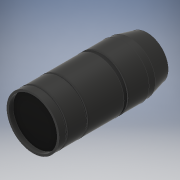
# Autodesk Inventor part: MLM3X-MP
Saved by Autodesk Inventor 2019 (Build 230136000, 136)
## iProperties
Created: 2019-03-17
Part Number: MLM3X-MP
Material: Acetal Resin, Black
Document SubType Name: Modeling
Designer: Wilson Lab
Density: 1.425 g/cm^3
Appearance: Smooth - Black
Author: Wilson Lab
Autodesk Inventor part; units mm, degrees
ref_plane "YZ Plane" through (0, 0, 0) normal (1, 0, 0) x (0, 1, 0)
ref_plane "XZ Plane" through (0, 0, 0) normal (0, 1, 0) x (-1, 0, 0)
ref_plane "XY Plane" through (0, 0, 0) normal (0, 0, 1) x (1, 0, 0)
sketch "Sketch1" plane through (0, 0, 0) normal (0, 0, 1) x (1, 0, 0)
  circle A0 centre (0, 0) radius 17.75
  dimension "d0" = 35.5
  constraints: 1 centre point, 1 coincident
  measures "d0" diameter of A0
extrude "Extrusion1" add sketch "Sketch1" along normal blind 16.8
sketch "Sketch2" plane through (0, 0, 16.8) normal (0, 0, 1) x (1, 0, 0)
  circle A0 centre (0, 0) radius 17.75 projected
  circle A1 centre (0, 0) radius 18.25
  dimension "d3" = 36.5
  constraints: 1 centre point, 1 coincident
  measures "d3" diameter of A1
extrude "Extrusion2" add sketch "Sketch2" along normal blind 14.7 contours A0 | A1
chamfer "Chamfer1" distance 3 distance2 12 1 edges at (-17.75, 0, 0) measured on face at (-0.7132, -5.1908, 0)
sketch "Sketch3" plane through (0, 0, 31.5) normal (0, 0, 1) x (1, 0, 0)
  circle A0 centre (0, 0) radius 18.25 projected
  circle A1 centre (0, 0) radius 17.75
  dimension "d9" = 35.5
  constraints: 1 centre point, 1 coincident
  measures "d9" diameter of A1
extrude "Extrusion3" add sketch "Sketch3" along normal blind 2.8 contours A1
sketch "Sketch4" plane through (0, 0, 34.3) normal (0, 0, 1) x (1, 0, 0)
  circle A0 centre (0, 0) radius 17.75 projected
  circle A1 centre (0, 0) radius 18.25
  dimension "d12" = 36.5
  constraints: 1 centre point, 1 coincident
  measures "d12" diameter of A1
extrude "Extrusion4" add sketch "Sketch4" along normal blind 25.25 contours A0 | A1
sketch "Sketch5" plane through (0, 0, 59.55) normal (0, 0, 1) x (1, 0, 0)
  circle A0 centre (0, 0) radius 18.25 projected
  circle A1 centre (0, 0) radius 17.75
  dimension "d15" = 35.5
  constraints: 1 centre point, 1 coincident
  measures "d15" diameter of A1
extrude "Extrusion5" add sketch "Sketch5" along normal blind 1 contours A1
sketch "Sketch6" plane through (0, 0, 60.55) normal (0, 0, 1) x (1, 0, 0)
  circle A0 centre (0, 0) radius 17.75 projected
  circle A1 centre (0, 0) radius 18.25
  dimension "d18" = 36.5
  constraints: 1 centre point, 1 coincident
  measures "d18" diameter of A1
extrude "Extrusion6" add sketch "Sketch6" along normal blind 13.2 contours A0 | A1
sketch "Sketch7" plane through (0, 0, 73.75) normal (0, 0, 1) x (1, 0, 0)
  circle A0 centre (0, 0) radius 18.25 projected
  circle A1 centre (0, 0) radius 17.75
  dimension "d21" = 35.5
  constraints: 1 centre point, 1 coincident
  measures "d21" diameter of A1
extrude "Extrusion7" add sketch "Sketch7" along normal blind 1 contours A1
sketch "Sketch8" plane through (0, 0, 74.75) normal (0, 0, 1) x (1, 0, 0)
  circle A0 centre (0, 0) radius 17.75 projected
  circle A1 centre (0, 0) radius 18.25
  dimension "d24" = 36.5
  constraints: 1 centre point, 1 coincident
  measures "d24" diameter of A1
extrude "Extrusion8" add sketch "Sketch8" along normal blind 4.85 contours A0 | A1
sketch "Sketch9" plane through (0, 0, 79.6) normal (0, 0, 1) x (1, 0, 0)
  circle A0 centre (0, 0) radius 16.9026
  constraints: 1 centre point, 1 coincident
extrude "Extrusion9" cut sketch "Sketch9" against normal blind 3
body "Solid1"
